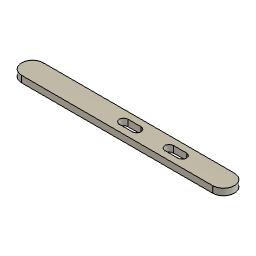
Encoder_Mount (Autodesk Fusion 360 design; units mm, degrees)
Autodesk Fusion 360 part; units mm, degrees
sketch "Sketch1" plane through (0, 0, 0) normal (0, 1, 0) x (1, 0, 0)
  line L0 (5, -5) -> (93, -5)
  arc A0 (93, -5) -> (93, 5) centre (93, 0) ccw
  line L1 (93, 5) -> (5, 5)
  arc A1 (5, 5) -> (5, -5) centre (5, 0) ccw
  line L2 (49, 5) -> (49, -5) construction
  line L3 (50, 0) -> (71, 0) construction
  line L4 (53, 2) -> (47, 2)
  arc A2 (47, 2) -> (47, -2) centre (47, 0) ccw
  line L5 (47, -2) -> (53, -2)
  arc A3 (53, -2) -> (53, 2) centre (53, 0) ccw
  line L6 (53, 0) -> (47, 0) construction
  line L7 (68, -2) -> (74, -2)
  arc A4 (74, -2) -> (74, 2) centre (74, 0) ccw
  line L8 (74, 2) -> (68, 2)
  arc A5 (68, 2) -> (68, -2) centre (68, 0) ccw
  line L9 (68, 0) -> (74, 0) construction
  point P0 (98, 0)
  point P1 (50, 0)
  point P2 (71, 0)
  point P3 (49, 0)
  dimension "d1" = 10
  dimension "d3" = 98
  dimension "d4" = 4
  dimension "d5" = 6
  dimension "d6" = 6
  dimension "d7" = 21
  dimension "d8" = 1
  constraint tangent L0 A0
  constraint tangent A0 L1
  constraint parallel L0 L1
  constraint tangent L1 A1
  constraint tangent L0 A1
  constraint midpoint A1 origin
  constraint midpoint A0 P0
  constraint horizontal origin P0
  constraint midpoint L1 L2.start
  constraint midpoint L0 L2.end
  constraint perpendicular L2 L3
  constraint tangent L4 A2
  constraint tangent A2 L5
  constraint parallel L4 L5
  constraint tangent L5 A3
  constraint tangent L4 A3
  constraint parallel L3 L6
  constraint coincident P1 L3.start
  constraint midpoint L6 P1
  constraint tangent L7 A4
  constraint tangent A4 L8
  constraint parallel L7 L8
  constraint tangent L8 A5
  constraint tangent L7 A5
  constraint parallel L4 L9
  constraint coincident P2 L3.end
  constraint midpoint L9 P2
  constraint equal A2 A5
  constraint midpoint L2 P3
  constraint coincident L3 P3
  measures "d1" diameter of A0
  measures "d3" horizontal distance of origin P0
  measures "d4" distance of L7 L8
  measures "d5" distance of A3.centre A2.centre
  measures "d6" distance of A5.centre A4.centre
  measures "d7" distance of P1 P2
  measures "d8" distance of L2 P1
extrude "Extrude1" add sketch "Sketch1" along normal blind 3
